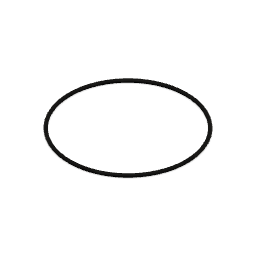
O ring 145 x 4 v2 (Autodesk Fusion 360 design; units mm, degrees)
Autodesk Fusion 360 part; units mm, degrees
sketch "Sketch1" plane through (0, 0, 0) normal (0, 0, 1) x (1, 0, 0)
  circle A0 centre (74.5, 0) radius 2
  dimension "d1" = 4
  dimension "d2" = 74.5
  constraint horizontal origin A0.centre
  measures "d1" diameter of A0
  measures "d2" horizontal distance of origin A0.centre
revolve "Revolve1" add sketch "Sketch1" angle 360 about axis through (0, 1.75, 0) along (0, 1, 0)
equation "d2 = ( 145 / 2 ) * 1 mm + 2 mm"
